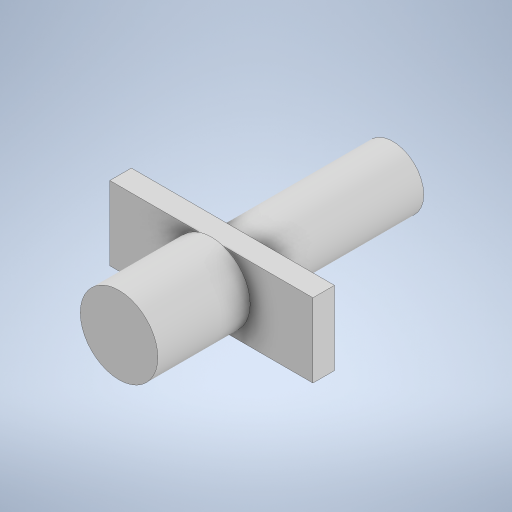
# Autodesk Inventor part: SMA whip end
Saved by Autodesk Inventor 2023 (Build 270158000, 158)
## iProperties
Created: 2023-01-23
Part Number: SMA whip end
Material: Generic
Document SubType Name: Modeling
Designer: Steven
Density: 1 g/cm^3
Appearance: Default
Author: Steven
Autodesk Inventor part; units mm, degrees
ref_plane "YZ Plane" through (0, 0, 0) normal (1, 0, 0) x (0, 1, 0)
ref_plane "XZ Plane" through (0, 0, 0) normal (0, 1, 0) x (-1, 0, 0)
ref_plane "XY Plane" through (0, 0, 0) normal (0, 0, 1) x (1, 0, 0)
sketch "Sketch1" plane through (0, 0, 0) normal (0, 0, 1) x (1, 0, 0)
  line L0 (0, 0) -> (35.3316, 0)
  line L1 (0, 0) -> (16.5, 0)
  line L2 (16.5, 0) -> (16.5, 6)
  line L3 (16.5, 6) -> (0, 6)
  line L4 (0, 6) -> (0, 0)
  dimension "d0" = 16.5
  dimension "d1" = 6
  constraints: 10 end point, 2 horizontal, 2 parallel, 1 perpendicular
  measures "d0" distance of L3.end L2.end
  measures "d1" distance of L2.end L1.end
extrude "Extrusion1" add sketch "Sketch1" along normal blind 1.75
sketch "Sketch2" plane through (0, 0, 1.75) normal (0, 0, 1) x (1, 0, 0)
  line L0 (0, 0) -> (16.5, 0) projected
  line L1 (16.5, 0) -> (16.5, 6) projected
  line L2 (16.5, 6) -> (0, 6) projected
  line L3 (0, 6) -> (0, 0) projected
  line L4 (8.25, 6) -> (8.25, 0) construction
  circle A0 centre (8.25, 3) radius 3.15
  dimension "d4" = 6.3
  constraints: 3 midpoint, 2 end point, 1 centre point
  measures "d4" diameter of A0
extrude "Extrusion2" add sketch "Sketch2" along normal blind 7.5 contours A0 L2 L0 | L0 A0 | A0 L2
sketch "Sketch3" plane through (0, 0, 0) normal (0, 0, -1) x (-1, 0, 0)
  line L0 (0, 0) -> (-16.5, 0) projected
  line L1 (0, 6) -> (0, 0) projected
  line L2 (-16.5, 6) -> (0, 6) projected
  line L3 (-16.5, 0) -> (-16.5, 6) projected
  line L4 (-8.25, 6) -> (-8.25, 0) construction
  circle A0 centre (-8.25, 3) radius 2.5
  dimension "d7" = 5
  constraints: 3 midpoint, 2 end point, 1 centre point
  measures "d7" diameter of A0
extrude "Extrusion3" add sketch "Sketch3" along normal blind 13 contours A0
body "Solid1"
